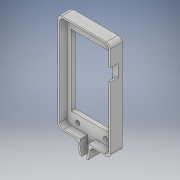
# Autodesk Inventor part: DS Phone Holder
Saved by Autodesk Inventor 2017 (Build 210142000, 142)
## iProperties
Created: 2019-01-26
Part Number: DS Phone Holder
Material: Generic
Document SubType Name: Modeling
Designer: Delta
Density: 1 g/cm^3
Appearance: Default
Author: Delta
Autodesk Inventor part; units mm, degrees
ref_plane "YZ Plane" through (0, 0, 0) normal (1, 0, 0) x (0, 1, 0)
ref_plane "XZ Plane" through (0, 0, 0) normal (0, 1, 0) x (-1, 0, 0)
sketch "Sketch1" plane through (0, 0, 0) normal (0, 0, 1) x (1, 0, 0)
  line L0 (0, 0) -> (81.28, 0)
  line L1 (81.28, 0) -> (81.28, 152.4)
  line L2 (81.28, 152.4) -> (0, 152.4)
  line L3 (0, 152.4) -> (0, 0)
  line L4 (8.89, 21.59) -> (72.39, 21.59)
  line L5 (72.39, 21.59) -> (72.39, 130.81)
  line L6 (72.39, 130.81) -> (8.89, 130.81)
  line L7 (8.89, 130.81) -> (8.89, 21.59)
  dimension "d0" = 81.28
  dimension "d1" = 152.4
  dimension "d2" = 21.59
  dimension "d3" = 8.89
  dimension "d4" = 63.5
  dimension "d5" = 109.22
  constraints: 16 end point, 4 parallel, 2 horizontal, 2 perpendicular
  measures "d0" distance of L2.end L1.end
  measures "d1" distance of L1.end L0.end
  measures "d2" distance from line of L0 L4.start
  measures "d3" distance from line of L3 L4.start
  measures "d4" distance of L6.end L5.end
  measures "d5" distance of L5.end L4.end
extrude "Extrusion1" add sketch "Sketch1" along normal blind 6.35
sketch "Sketch2" plane through (0, 0, 6.35) normal (0, 0, 1) x (1, 0, 0)
  line L0 (0, 0) -> (81.28, 0)
  line L1 (81.28, 0) -> (81.28, 152.4)
  line L2 (81.28, 152.4) -> (0, 152.4)
  line L3 (0, 152.4) -> (0, 0)
  line L4 (2.54, 2.54) -> (78.74, 2.54)
  line L5 (78.74, 2.54) -> (78.74, 149.86)
  line L6 (78.74, 149.86) -> (2.54, 149.86)
  line L7 (2.54, 149.86) -> (2.54, 2.54)
  dimension "d8" = 2.54
  dimension "d9" = 2.54
  dimension "d10" = 76.2
  dimension "d11" = 147.32
  constraints: 16 end point, 4 parallel, 2 horizontal, 2 perpendicular
  measures "d8" distance from line of L4.start L0
  measures "d9" distance from line of L3 L4.start
  measures "d10" distance of L6.end L5.end
  measures "d11" distance of L5.end L4.end
extrude "Extrusion2" add sketch "Sketch2" along normal blind 11.684
sketch "Sketch3" plane through (0, 0, 18.034) normal (0, 0, 1) x (1, 0, 0)
  line L0 (0, 0) -> (81.28, 0) projected
  line L1 (2.54, 2.54) -> (78.74, 2.54) projected
  line L2 (34.29, 0) -> (46.99, 0)
  line L3 (46.99, 0) -> (46.99, 2.54)
  line L4 (46.99, 2.54) -> (34.29, 2.54)
  line L5 (34.29, 2.54) -> (34.29, 0)
  line L6 (81.28, 0) -> (81.28, 152.4) projected
  line L7 (81.28, 152.4) -> (0, 152.4) projected
  line L8 (78.74, 2.54) -> (78.74, 149.86) projected
  line L9 (81.28, 121.285) -> (78.74, 121.285)
  line L10 (78.74, 121.285) -> (78.74, 102.235)
  line L11 (78.74, 102.235) -> (81.28, 102.235)
  line L12 (81.28, 102.235) -> (81.28, 121.285)
  dimension "d14" = 34.29
  dimension "d15" = 12.7
  dimension "d16" = 31.115
  dimension "d17" = 19.05
  constraints: 16 end point, 4 parallel, 4 point on line, 2 horizontal, 2 perpendicular
  measures "d14" distance of L0.start L2.start
  measures "d15" distance of L4.end L3.end
  measures "d16" distance from line of L7 L9.start
  measures "d17" distance of L10.end L9.end
extrude "Extrusion3" cut sketch "Sketch3" against normal blind 11.684 contours L5 L1 L3 L0 | L11 L8 L9 L6
fillet "Fillet1" radius 6.35 1 edges at (78.74, 149.86, 12.192)
fillet "Fillet2" radius 6.35 3 edges at (2.54, 149.86, 12.192) (2.54, 2.54, 12.192) (78.74, 2.54, 12.192)
fillet "Fillet3" radius 6.35 4 edges at (81.28, 0, 9.017) (0, 0, 9.017) (81.28, 152.4, 9.017) (0, 152.4, 9.017)
sketch "Sketch4" plane through (0, 0, 0) normal (0, 0, -1) x (-1, 0, 0)
  line L0 (-46.99, 0) -> (-34.29, 0) projected
  arc A0 (-37.465, -19.05) -> (-34.29, 0) centre (-72.232, -3.4659) ccw
  arc A1 (-46.99, 0) -> (-43.815, -19.05) centre (-9.048, -3.4659) ccw
  line L1 (-6.35, 0) -> (-34.29, 0) projected
  line L2 (-6.35, 0) -> (-74.93, 0) projected
  arc A2 (-34.29, -19.05) -> (-31.75, 0) centre (-69.5649, -4.6523) ccw
  arc A3 (-49.53, 0) -> (-46.6296, -19.05) centre (-11.6381, -3.9766) ccw
  line L3 (-34.29, -19.05) -> (-37.465, -19.05)
  line L4 (-46.6296, -19.05) -> (-43.815, -19.05)
  point P0 (0, 0)
  dimension "d24" = 19.05
  dimension "d25" = 3.175
  dimension "d26" = 3.175
  dimension "d27" = 38.1
  dimension "d28" = 38.1
  dimension "d29" = 2.54
  dimension "d30" = 2.54
  dimension "d31" = 38.1
  dimension "d32" = 38.1
  dimension "d33" = 3.175
  constraints: 8 point on circle, 4 centre point, 4 end point, 2 point on line, 1 collinear, 1 horizontal
  measures "d24" vertical distance of L4.end L0.start
  measures "d25" horizontal distance of L3.end L0.end
  measures "d26" horizontal distance of L4.end L0.start
  measures "d27" radius of A0
  measures "d28" radius of A1
  measures "d29" distance of L0.end A2.end
  measures "d30" distance of A3.start L0.start
  measures "d31" radius of A2
  measures "d32" radius of A3
  measures "d33" distance of L3.start L3.end
extrude "Extrusion4" add sketch "Sketch4" against normal blind 18.034
fillet "Fillet4" radius 6.35 1 edges at (31.75, 0, 9.017)
fillet "Fillet5" radius 6.35 1 edges at (49.53, 0, 9.017)
sketch "Sketch5" plane through (0, 0, 0) normal (0, 0, -1) x (-1, 0, 0)
  arc A0 (-35.9722, -19.0303) -> (-32.9017, 0) centre (-116.0568, 3.6542) ccw
  arc A1 (-49.1616, 0) -> (-45.6026, -19.0303) centre (-4.2841, -1.455) ccw
  arc A2 (-32.9017, 0) -> (-49.1616, 0) centre (-41.0317, -15.216) ccw
  line L0 (-35.9722, -19.0303) -> (-45.6026, -19.0303)
  line L1 (-46.6296, -19.05) -> (-43.815, -19.05) projected
  point P0 (0, 0)
  constraints: 6 point on circle, 3 centre point, 2 end point, 1 parallel
extrude "Extrusion5" add sketch "Sketch5" against normal blind 6.35
sketch "Sketch6" plane through (0, 0, 6.35) normal (0, 0, 1) x (1, 0, 0)
  line L0 (74.93, 152.4) -> (6.35, 152.4) projected
  line L1 (6.35, 0) -> (25.1473, 0) projected
  line L2 (0, 146.05) -> (0, 6.35) projected
  point P0 (0, 0)
  point P1 (19.05, 10.795)
  point P2 (19.05, 141.605)
  dimension "d40" = 10.795
  dimension "d41" = 10.795
  dimension "d42" = 19.05
  dimension "d43" = 19.05
  measures "d40" distance from line of L0 point (19.05, 141.605)
  measures "d41" distance from line of L1 point (19.05, 10.795)
  measures "d42" distance from line of L2 point (19.05, 141.605)
  measures "d43" distance from line of L2 point (19.05, 10.795)
hole "Hole1" at (19.05, 10.795, 6.35) at (19.05, 141.605, 6.35) direction (0, 0, -1) diameter 3.683 depth 25.4 tip angle 118
sketch "Sketch7" plane through (0, 0, 6.35) normal (0, 0, 1) x (1, 0, 0)
  circle A0 centre (19.05, 10.795) radius 1.8415 projected
  circle A1 centre (19.05, 10.795) radius 3.4925
  circle A2 centre (19.05, 141.605) radius 1.8415 projected
  circle A3 centre (19.05, 141.605) radius 3.4925
  point P0 (0, 0)
  dimension "d51" = 6.985
  dimension "d52" = 6.985
  constraints: 2 centre point, 2 coincident
  measures "d51" diameter of A1
  measures "d52" diameter of A3
extrude "Extrusion6" cut sketch "Sketch7" against normal blind 2.54
ref_plane "Work Plane1" through (40.64, 102.235, 6.35) normal (1, 0, 0) x (0, 0, -1)
mirror "Mirror1" about plane through (40.64, 102.235, 6.35) normal (1, 0, 0) of "Extrusion6", "Hole1"
equation "\"d26\" = d25"
equation "\"d28\" = d27"
equation "\"d30\" = d29"
body "Solid1"
